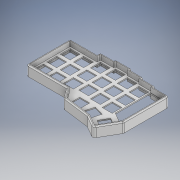
# Autodesk Inventor part: imk
Saved by Autodesk Inventor 2021 (Build 250183000, 183)
## iProperties
Created: 2022-05-13
Part Number: imk
Material: Generic
Document SubType Name: Modeling
Designer: Mark
Density: 1 g/cm^3
Appearance: Default
Author: Mark
Autodesk Inventor part; units mm, degrees
ref_plane "YZ Plane" through (0, 0, 0) normal (1, 0, 0) x (0, 1, 0)
ref_plane "XZ Plane" through (0, 0, 0) normal (0, 1, 0) x (-1, 0, 0)
ref_plane "XY Plane" through (0, 0, 0) normal (0, 0, 1) x (1, 0, 0)
sketch "keyholes" plane through (0, 0, 0) normal (0, 0, 1) x (1, 0, 0)
  line L0 (76.8681, -69.6062) -> (62.8681, -69.6062)
  line L1 (62.8681, -69.6062) -> (62.8681, -55.6062)
  line L2 (62.8681, -55.6062) -> (76.8681, -55.6062)
  line L3 (76.8681, -55.6062) -> (76.8681, -69.6062)
  line L4 (76.8681, -50.6062) -> (62.8681, -50.6062)
  line L5 (62.8681, -50.6062) -> (62.8681, -36.6062)
  line L6 (62.8681, -36.6062) -> (76.8681, -36.6062)
  line L7 (76.8681, -36.6062) -> (76.8681, -50.6062)
  line L8 (76.8681, -31.6062) -> (62.8681, -31.6062)
  line L9 (62.8681, -31.6062) -> (62.8681, -17.6062)
  line L10 (62.8681, -17.6062) -> (76.8681, -17.6062)
  line L11 (76.8681, -17.6062) -> (76.8681, -31.6062)
  point P0 (69.8681, -43.6062)
  dimension "d0" = 14
  dimension "d1" = 14
  dimension "d2" = 14
  dimension "d3" = 14
  dimension "d4" = 14
  dimension "d5" = 14
  dimension "d6" = 5
  dimension "d7" = 5
  measures "d0" distance of L1.end L2.end
  measures "d1" distance of L0.end L1.end
  measures "d2" distance of L5.end L6.end
  measures "d3" distance of L4.end L5.end
  measures "d4" distance of L9.end L10.end
  measures "d5" distance of L8.end L9.end
  measures "d6" distance between parallel lines of L4 L2
  measures "d7" distance between parallel lines of L8 L6
sketch "Sketch1" plane through (0, 0, 0) normal (0, 1, 0) x (-1, 0, 0)
  line L0 (119.155, -84.8943) -> (82.155, -84.8943)
  line L1 (64.1602, -28.6437) -> (119.155, -28.6437)
  line L2 (119.655, -29.1437) -> (119.655, -84.3943)
  line L3 (81.655, -85.3943) -> (81.655, -89.1443)
  line L4 (81.155, -89.6443) -> (63.155, -89.6443)
  line L5 (62.655, -90.1443) -> (62.655, -91.3943)
  line L6 (62.155, -91.8943) -> (45.155, -91.8943)
  line L7 (44.655, -91.3943) -> (44.655, -90.1443)
  line L8 (44.155, -89.6443) -> (26.155, -89.6443)
  line L9 (25.655, -89.1443) -> (25.655, -87.645)
  line L10 (25.155, -87.145) -> (7.155, -87.145)
  line L11 (63.7562, -28.4383) -> (53.3017, -14.1027)
  line L12 (52.9623, -13.9015) -> (15.7765, -9.0643)
  line L13 (15.591, -9.0015) -> (0.433, -0.25)
  line L14 (-0.25, -0.433) -> (-13.766, -23.8434)
  line L15 (-13.766, -23.8434) -> (6.655, -35.6335)
  line L16 (51.1256, -15.8625) -> (37.1256, -15.8625)
  line L17 (37.1256, -15.8625) -> (37.1256, -29.8625)
  line L18 (37.1256, -29.8625) -> (51.1256, -29.8625)
  line L19 (51.1256, -29.8625) -> (51.1256, -15.8625)
  line L20 (28.1127, -28.7255) -> (14.5898, -25.1021)
  line L21 (14.5898, -25.1021) -> (18.2132, -11.5791)
  line L22 (18.2132, -11.5791) -> (31.7362, -15.2026)
  line L23 (31.7362, -15.2026) -> (28.1127, -28.7255)
  line L24 (6.155, -84.895) -> (-13.5994, -84.895)
  line L25 (-14.0994, -84.395) -> (-14.0994, -24.5548)
  line L26 (-13.766, -23.8434) -> (-14.0324, -24.3048)
  line L27 (3.4672, -25.9744) -> (-8.6572, -18.9744)
  line L28 (-8.6572, -18.9744) -> (-1.6572, -6.85)
  line L29 (-1.6572, -6.85) -> (10.4672, -13.85)
  line L30 (10.4672, -13.85) -> (3.4672, -25.9744)
  arc A0 (119.155, -84.8943) -> (119.655, -84.3943) centre (119.155, -84.3943) ccw
  arc A1 (82.155, -84.8943) -> (81.655, -85.3943) centre (82.155, -85.3943) ccw
  arc A2 (81.155, -89.6443) -> (81.655, -89.1443) centre (81.155, -89.1443) ccw
  arc A3 (62.155, -91.8943) -> (62.655, -91.3943) centre (62.155, -91.3943) ccw
  arc A4 (44.655, -90.1443) -> (44.155, -89.6443) centre (44.155, -90.1443) ccw
  arc A5 (44.655, -91.3943) -> (45.155, -91.8943) centre (45.155, -91.3943) ccw
  arc A6 (63.155, -89.6443) -> (62.655, -90.1443) centre (63.155, -90.1443) ccw
  arc A7 (25.655, -89.1443) -> (26.155, -89.6443) centre (26.155, -89.1443) ccw
  arc A8 (-14.0994, -84.395) -> (-13.5994, -84.895) centre (-13.5994, -84.395) ccw
  line L31 (6.655, -86.645) -> (6.655, -85.395)
  arc A9 (25.655, -87.645) -> (25.155, -87.145) centre (25.155, -87.645) ccw
  arc A10 (6.655, -86.645) -> (7.155, -87.145) centre (7.155, -86.645) ccw
  arc A11 (6.655, -85.395) -> (6.155, -84.895) centre (6.155, -85.395) ccw
  arc A12 (-14.0324, -24.3048) -> (-14.0994, -24.5548) centre (-13.5994, -24.5548) ccw
  arc A13 (0.433, -0.25) -> (-0.25, -0.433) centre (0.183, -0.683) ccw
  arc A14 (15.591, -9.0015) -> (15.7765, -9.0643) centre (15.841, -8.5685) ccw
  arc A15 (53.3017, -14.1027) -> (52.9623, -13.9015) centre (52.8978, -14.3973) ccw
  arc A16 (63.7562, -28.4383) -> (64.1602, -28.6437) centre (64.1602, -28.1437) ccw
  arc A17 (119.655, -29.1437) -> (119.155, -28.6437) centre (119.155, -29.1437) ccw
  line L32 (84.655, -87.8943) -> (119.155, -87.8943)
  arc A18 (119.155, -87.8943) -> (122.655, -84.3943) centre (119.155, -84.3943) ccw
  line L33 (122.655, -84.3943) -> (122.655, -29.1437)
  arc A19 (122.655, -29.1437) -> (119.155, -25.6437) centre (119.155, -29.1437) ccw
  line L34 (119.155, -25.6437) -> (65.4312, -25.6437)
  line L35 (65.4312, -25.6437) -> (55.7257, -12.335)
  arc A20 (55.7257, -12.335) -> (53.3492, -10.9266) centre (52.8978, -14.3973) ccw
  line L36 (53.3492, -10.9266) -> (16.6586, -6.1538)
  line L37 (16.6586, -6.1538) -> (1.933, 2.3481)
  arc A21 (1.933, 2.3481) -> (-2.8481, 1.067) centre (0.183, -0.683) ccw
  line L38 (-2.8481, 1.067) -> (-16.3641, -22.3434)
  line L39 (-16.3641, -22.3434) -> (-16.6305, -22.8048)
  arc A22 (-16.6305, -22.8048) -> (-17.0994, -24.5548) centre (-13.5994, -24.5548) ccw
  line L40 (-17.0994, -24.5548) -> (-17.0994, -84.395)
  arc A23 (-17.0994, -84.395) -> (-13.5994, -87.895) centre (-13.5994, -84.395) ccw
  line L41 (-13.5994, -87.895) -> (3.8858, -87.895)
  arc A24 (3.8858, -87.895) -> (7.155, -90.145) centre (7.155, -86.645) ccw
  line L42 (7.155, -90.145) -> (22.8011, -90.145)
  arc A25 (22.8011, -90.145) -> (26.155, -92.6443) centre (26.155, -89.1443) ccw
  line L43 (26.155, -92.6443) -> (41.8858, -92.6443)
  arc A26 (41.8858, -92.6443) -> (45.155, -94.8943) centre (45.155, -91.3943) ccw
  line L44 (45.155, -94.8943) -> (62.155, -94.8943)
  arc A27 (62.155, -94.8943) -> (65.4242, -92.6443) centre (62.155, -91.3943) ccw
  line L45 (65.4242, -92.6443) -> (81.155, -92.6443)
  arc A28 (81.155, -92.6443) -> (84.655, -89.1443) centre (81.155, -89.1443) ccw
  line L46 (84.655, -89.1443) -> (84.655, -87.8943)
  line L47 (82.155, -85.3943) -> (119.155, -85.3943)
  arc A29 (119.155, -85.3943) -> (120.155, -84.3943) centre (119.155, -84.3943) ccw
  line L48 (120.155, -84.3943) -> (120.155, -29.1437)
  arc A30 (120.155, -29.1437) -> (119.155, -28.1437) centre (119.155, -29.1437) ccw
  line L49 (119.155, -28.1437) -> (64.1602, -28.1437)
  line L50 (64.1602, -28.1437) -> (53.7057, -13.8081)
  arc A31 (53.7057, -13.8081) -> (53.0268, -13.4057) centre (52.8978, -14.3973) ccw
  line L51 (53.0268, -13.4057) -> (15.841, -8.5685)
  line L52 (15.841, -8.5685) -> (0.683, 0.183)
  arc A32 (0.683, 0.183) -> (-0.683, -0.183) centre (0.183, -0.683) ccw
  line L53 (-0.683, -0.183) -> (-14.199, -23.5934)
  line L54 (-14.199, -23.5934) -> (-14.4654, -24.0548)
  arc A33 (-14.4654, -24.0548) -> (-14.5994, -24.5548) centre (-13.5994, -24.5548) ccw
  line L55 (-14.5994, -24.5548) -> (-14.5994, -84.395)
  arc A34 (-14.5994, -84.395) -> (-13.5994, -85.395) centre (-13.5994, -84.395) ccw
  line L56 (-13.5994, -85.395) -> (6.155, -85.395)
  line L57 (6.155, -85.395) -> (6.155, -86.645)
  arc A35 (6.155, -86.645) -> (7.155, -87.645) centre (7.155, -86.645) ccw
  line L58 (7.155, -87.645) -> (25.155, -87.645)
  line L59 (25.155, -87.645) -> (25.155, -89.1443)
  arc A36 (25.155, -89.1443) -> (26.155, -90.1443) centre (26.155, -89.1443) ccw
  line L60 (26.155, -90.1443) -> (44.155, -90.1443)
  line L61 (44.155, -90.1443) -> (44.155, -91.3943)
  arc A37 (44.155, -91.3943) -> (45.155, -92.3943) centre (45.155, -91.3943) ccw
  line L62 (45.155, -92.3943) -> (62.155, -92.3943)
  arc A38 (62.155, -92.3943) -> (63.155, -91.3943) centre (62.155, -91.3943) ccw
  line L63 (63.155, -91.3943) -> (63.155, -90.1443)
  line L64 (63.155, -90.1443) -> (81.155, -90.1443)
  arc A39 (81.155, -90.1443) -> (82.155, -89.1443) centre (81.155, -89.1443) ccw
  line L65 (82.155, -89.1443) -> (82.155, -85.3943)
  line L66 (6.655, -35.6335) -> (6.655, -85.395)
  line L67 (98.644, -82.7713) -> (84.644, -82.7713)
  line L68 (84.644, -82.7713) -> (84.644, -68.7713)
  line L69 (84.644, -68.7713) -> (98.644, -68.7713)
  line L70 (98.644, -68.7713) -> (98.644, -82.7713)
  line L71 (98.644, -63.7713) -> (84.644, -63.7713)
  line L72 (84.644, -63.7713) -> (84.644, -49.7713)
  line L73 (84.644, -49.7713) -> (98.644, -49.7713)
  line L74 (98.644, -49.7713) -> (98.644, -63.7713)
  line L75 (98.644, -44.7713) -> (84.644, -44.7713)
  line L76 (84.644, -44.7713) -> (84.644, -30.7713)
  line L77 (84.644, -30.7713) -> (98.644, -30.7713)
  line L78 (98.644, -30.7713) -> (98.644, -44.7713)
  line L79 (117.644, -82.7713) -> (103.644, -82.7713)
  line L80 (103.644, -82.7713) -> (103.644, -68.7713)
  line L81 (103.644, -68.7713) -> (117.644, -68.7713)
  line L82 (117.644, -68.7713) -> (117.644, -82.7713)
  line L83 (117.644, -63.7713) -> (103.644, -63.7713)
  line L84 (103.644, -63.7713) -> (103.644, -49.7713)
  line L85 (103.644, -49.7713) -> (117.644, -49.7713)
  line L86 (117.644, -49.7713) -> (117.644, -63.7713)
  line L87 (117.644, -44.7713) -> (103.644, -44.7713)
  line L88 (103.644, -44.7713) -> (103.644, -30.7713)
  line L89 (103.644, -30.7713) -> (117.644, -30.7713)
  line L90 (117.644, -30.7713) -> (117.644, -44.7713)
  line L91 (79.644, -87.5161) -> (65.644, -87.5161)
  line L92 (65.644, -87.5161) -> (65.644, -73.5161)
  line L93 (65.644, -73.5161) -> (79.644, -73.5161)
  line L94 (79.644, -73.5161) -> (79.644, -87.5161)
  line L95 (79.644, -68.5161) -> (65.644, -68.5161)
  line L96 (65.644, -68.5161) -> (65.644, -54.5161)
  line L97 (65.644, -54.5161) -> (79.644, -54.5161)
  line L98 (79.644, -54.5161) -> (79.644, -68.5161)
  line L99 (79.644, -49.5161) -> (65.644, -49.5161)
  line L100 (65.644, -49.5161) -> (65.644, -35.5161)
  line L101 (65.644, -35.5161) -> (79.644, -35.5161)
  line L102 (79.644, -35.5161) -> (79.644, -49.5161)
  line L103 (60.644, -89.895) -> (46.644, -89.895)
  line L104 (46.644, -89.895) -> (46.644, -75.895)
  line L105 (46.644, -75.895) -> (60.644, -75.895)
  line L106 (60.644, -75.895) -> (60.644, -89.895)
  line L107 (60.644, -70.895) -> (46.644, -70.895)
  line L108 (46.644, -70.895) -> (46.644, -56.895)
  line L109 (46.644, -56.895) -> (60.644, -56.895)
  line L110 (60.644, -56.895) -> (60.644, -70.895)
  line L111 (60.644, -51.895) -> (46.644, -51.895)
  line L112 (46.644, -51.895) -> (46.644, -37.895)
  line L113 (46.644, -37.895) -> (60.644, -37.895)
  line L114 (60.644, -37.895) -> (60.644, -51.895)
  line L115 (41.644, -87.5204) -> (27.644, -87.5204)
  line L116 (27.644, -87.5204) -> (27.644, -73.5204)
  line L117 (27.644, -73.5204) -> (41.644, -73.5204)
  line L118 (41.644, -73.5204) -> (41.644, -87.5204)
  line L119 (41.644, -68.5204) -> (27.644, -68.5204)
  line L120 (27.644, -68.5204) -> (27.644, -54.5204)
  line L121 (27.644, -54.5204) -> (41.644, -54.5204)
  line L122 (41.644, -54.5204) -> (41.644, -68.5204)
  line L123 (41.644, -49.5204) -> (27.644, -49.5204)
  line L124 (27.644, -49.5204) -> (27.644, -35.5204)
  line L125 (27.644, -35.5204) -> (41.644, -35.5204)
  line L126 (41.644, -35.5204) -> (41.644, -49.5204)
  line L127 (22.644, -85.1356) -> (8.644, -85.1356)
  line L128 (8.644, -85.1356) -> (8.644, -71.1356)
  line L129 (8.644, -71.1356) -> (22.644, -71.1356)
  line L130 (22.644, -71.1356) -> (22.644, -85.1356)
  line L131 (22.644, -66.1356) -> (8.644, -66.1356)
  line L132 (8.644, -66.1356) -> (8.644, -52.1356)
  line L133 (8.644, -52.1356) -> (22.644, -52.1356)
  line L134 (22.644, -52.1356) -> (22.644, -66.1356)
  line L135 (22.644, -47.1356) -> (8.644, -47.1356)
  line L136 (8.644, -47.1356) -> (8.644, -33.1356)
  line L137 (8.644, -33.1356) -> (22.644, -33.1356)
  line L138 (22.644, -33.1356) -> (22.644, -47.1356)
  point P0 (119.655, -84.8943)
  point P1 (63.906, -28.6437)
  point P2 (81.655, -84.8943)
  point P3 (119.655, -28.6437)
  point P4 (81.655, -89.6443)
  point P5 (62.655, -89.6443)
  point P6 (62.655, -91.8943)
  point P7 (44.655, -91.8943)
  point P8 (44.655, -89.6443)
  point P9 (25.655, -89.6443)
  point P10 (25.655, -87.145)
  point P11 (53.1752, -13.9292)
  point P12 (15.6775, -9.0514)
  point P13 (0, 0)
  point P14 (-14.0994, -84.895)
  point P15 (0, 0)
  point P16 (6.655, -87.145)
  dimension "d8" = 5
  dimension "d14" = 4.7448
  dimension "d15" = 5
  dimension "d18" = 2.3788
  dimension "d19" = 5
  dimension "d22" = 5
  dimension "d23" = 5
  dimension "d24" = 2.3746
  dimension "d25" = 2.3849
  dimension "d9" = 2.123
  dimension "d10" = 2.011
  dimension "d11" = 38
  dimension "d12" = 4.75
  dimension "d13" = 2.1277
  dimension "d16" = 19
  dimension "d17" = 2.25
  dimension "d20" = 18
  dimension "d21" = 2.25
  dimension "d26" = 19
  dimension "d27" = 19
  dimension "d28" = 55.749
  dimension "d29" = 18.2117
  dimension "d30" = 126.102
  dimension "d31" = 133.514
  dimension "d32" = 37.8137
  dimension "d33" = 18.1028
  dimension "d37" = 27.532
  dimension "d39" = 14
  dimension "d40" = 14
  dimension "d41" = 5.6579
  dimension "d42" = 4.5184
  dimension "d43" = 14
  dimension "d44" = 14
  dimension "d45" = 15
  dimension "d46" = 5.3894
  dimension "d47" = 1.137
  dimension "d48" = 2.25
  dimension "d50" = 14
  dimension "d51" = 14
  dimension "d52" = 30
  dimension "d53" = 7.7461
  dimension "d54" = 11.2521
  dimension "d55" = 90
  dimension "d56" = 90
  dimension "d58" = 2.4994
  dimension "d59" = 0.5
  dimension "d60" = 0.5
  dimension "d66" = 0.5
  dimension "d67" = 0.5
  dimension "d68" = 20.7543
  dimension "d69" = 3
  dimension "d70" = 0.5
  constraints: 134 end point, 80 point on circle, 40 centre point, 36 tangent, 32 point on line, 16 perpendicular, 14 equal radius, 10 parallel, 4 horizontal, 4 vertical, 3 collinear, 1 coincident, 54 other
  measures "d11" distance of point (119.655, -84.894) point (81.655, -84.894)
  measures "d12" distance of point (81.655, -84.894) point (81.655, -89.644)
  measures "d16" distance of point (81.655, -89.644) point (62.655, -89.644)
  measures "d17" distance between parallel lines of L6 L4
  measures "d20" distance of point (62.655, -91.894) point (44.655, -91.894)
  measures "d21" distance of point (44.655, -91.894) point (44.655, -89.644)
  measures "d26" distance of point (44.655, -89.644) point (25.655, -89.644)
  measures "d27" distance of point (6.655, -87.145) point (25.655, -87.145)
  measures "d28" distance of point (63.906, -28.644) point (119.655, -28.644)
  measures "d29" distance of point (63.906, -28.644) point (53.175, -13.929)
  measures "d30" angle of L11 L1
  measures "d31" angle of L12 L11
  measures "d32" distance of point (53.175, -13.929) point (15.677, -9.051)
  measures "d33" distance of point (15.677, -9.051) point (0, 0)
  measures "d37" distance of point (0, 0) L14.end
  measures "d39" distance of L18.end L17.end
  measures "d40" distance of L17.end L16.end
  measures "d43" distance of L21.end L22.end
  measures "d44" distance of L20.end L21.end
  measures "d45" angle of L23 L17
  measures "d46" horizontal distance of L22.end L16.end
  measures "d47" vertical distance of L20.start L17.end
  measures "d48" distance between parallel lines of L24 L10
  measures "d50" distance of L28.end L29.end
  measures "d51" distance of L28.start L28.end
  measures "d52" angle of L17 L30
  measures "d53" horizontal distance of L29.end L21.end
  measures "d54" vertical distance of L29.end L20.end
  measures "d55" angle of L14 L13
  measures "d56" angle of L15 L14
  measures "d58" distance of point (25.655, -89.644) point (25.655, -87.145)
  measures "d59" radius of A0
  measures "d60" radius of A3
  measures "d66" radius of A9
  measures "d67" radius of A8
  measures "d68" distance between parallel lines of L25 L31
  measures "d69" distance between parallel lines of L0 L32
  measures "d70" distance between parallel lines of L0 L47
extrude "Extrusion1" add sketch "Sketch1" along normal blind 1.5 contours L0 A1 L3 A2 L4 A6 L5 A3 L6 A5 L7 A4 L8 A7 L9 A9 L10 A10 L31 L66 L15 L14 A13 L13 A14 L12 A15 L11 A16 L1 A17 L2 A0 | L65 A39 L64 L63 A38 L62 A37 L61 L60 A36 L59 L58 A35 L57 L56 A34 L55 A33 L54 L53 A32 L52 L51 A31 L50 L49 A30 L48 A29 L47
extrude "Extrusion2" add sketch "Sketch1" along normal blind 8.5 and the other way blind 5.5 contours L46 A28 L45 A27 L44 A26 L43 A25 L42 A24 L41 A23 L40 A22 L39 L38 A21 L37 L36 A20 L35 L34 A19 L33 A18 L32
chamfer "Chamfer1" distance 1.5 angle 45 26 edges at (-92.2931, 8.5, -25.6437) (-121.6299, 8.5, -26.6688) (-122.655, 8.5, -56.769) (-121.6299, 8.5, -86.8692) (-101.905, 8.5, -87.8943) (-60.5784, 8.5, -18.9893) (-54.6823, 8.5, -11.3864) (-35.0039, 8.5, -8.5402) (-9.2958, 8.5, -1.9028) (0.7229, 8.5, 2.6977) (9.6061, 8.5, -10.6382) (16.4973, 8.5, -22.5741) (16.9801, 8.5, -23.6489) (17.0994, 8.5, -54.4749) (16.0742, 8.5, -86.8698) (4.8568, 8.5, -87.895) (-14.978, 8.5, -90.145) (-5.1707, 8.5, -89.5281) (-34.0204, 8.5, -92.6443) (-24.0636, 8.5, -91.9508) (-53.655, 8.5, -94.8943) (-64.1393, 8.5, -94.2775) (-43.1707, 8.5, -94.2775) (-73.2896, 8.5, -92.6443) (-83.6299, 8.5, -91.6192) (-84.655, 8.5, -88.5193)
body "Solid1"
